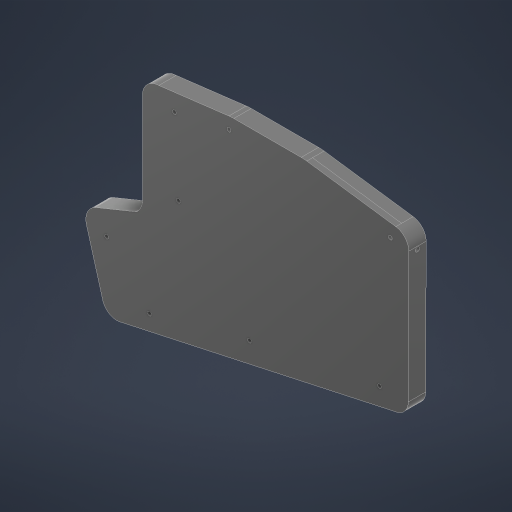
# Autodesk Inventor part: Case Bottom
Saved by Autodesk Inventor 2024.3 (Build 283343000, 343)
## iProperties
Created: 2024-12-13
Part Number: Case Bottom
Material: Generic
Document SubType Name: Modeling
Designer: micha
Density: 1 g/cm^3
Appearance: Smooth - Black
Author: micha
Autodesk Inventor part; units mm, degrees
ref_plane "YZ Plane" through (0, 0, 0) normal (1, 0, 0) x (0, 1, 0)
ref_plane "XZ Plane" through (0, 0, 0) normal (0, 1, 0) x (-1, 0, 0)
ref_plane "XY Plane" through (0, 0, 0) normal (0, 0, 1) x (1, 0, 0)
sketch "Sketch1" plane through (0, 0, 0) normal (0, 0, 1) x (1, 0, 0)
  arc A0 (-212.539, -59.4694) -> (-218.5045, -64.8588) centre (-212.5401, -65.4644) ccw projected
  line L0 (-174.0364, -54.7609) -> (-212.539, -59.4694) projected
  arc A1 (-171.7239, -54.62) -> (-174.0364, -54.7609) centre (-171.7239, -73.6702) ccw projected
  line L1 (-134.8832, -54.62) -> (-171.7239, -54.62) projected
  arc A2 (-132.2802, -54.7987) -> (-134.8832, -54.62) centre (-134.8832, -73.6711) ccw projected
  line L2 (-83.5422, -61.5211) -> (-132.2802, -54.7987) projected
  arc A3 (-79.23, -66.4736) -> (-83.5422, -61.5211) centre (-84.23, -66.4736) ccw projected
  line L3 (-79.4773, -138.0224) -> (-79.23, -66.4736) projected
  arc A4 (-82.9877, -142.7953) -> (-79.4773, -138.0224) centre (-84.4773, -138.0223) ccw projected
  line L4 (-234.3607, -175.7237) -> (-82.9877, -142.7953) projected
  arc A5 (-240.2338, -172.8773) -> (-234.3607, -175.7237) centre (-235.7454, -171.0986) ccw projected
  line L5 (-249.3284, -140.9769) -> (-240.2338, -172.8773) projected
  arc A6 (-246.2558, -134.3964) -> (-249.3284, -140.9769) centre (-243.557, -139.6641) ccw projected
  line L6 (-224.2532, -125.4096) -> (-246.2558, -134.3964) projected
  arc A7 (-224.2532, -125.4096) -> (-221.4228, -123.1302) centre (-226.6543, -119.531) ccw projected
  line L7 (-220.6818, -122.0531) -> (-221.4228, -123.1302) projected
  arc A8 (-220.6818, -122.0531) -> (-218.4447, -114.8395) centre (-231.1445, -114.8548) ccw projected
  line L8 (-218.5045, -64.8588) -> (-218.4447, -114.8395) projected
  circle A9 centre (-163.195, -152.4) radius 1.05 projected
  circle A10 centre (-92.075, -138.43) radius 1.05 projected
  circle A11 centre (-86.11, -127.04) radius 0.8509 projected
  circle A12 centre (-91.61, -127.04) radius 1.7145 projected
  circle A13 centre (-97.11, -127.04) radius 0.8509 projected
  circle A14 centre (-104.11, -127.04) radius 0.8509 projected
  circle A15 centre (-122.11, -139.04) radius 0.8509 projected
  circle A16 centre (-122.61, -135.29) radius 1.5 projected
  circle A17 centre (-109.61, -127.04) radius 1.7145 projected
  circle A18 centre (-115.11, -127.04) radius 0.8509 projected
  circle A19 centre (-86.61, -123.29) radius 1.5 projected
  circle A20 centre (-91.61, -121.09) radius 1.5 projected
  circle A21 centre (-96.61, -123.29) radius 1.5 projected
  circle A22 centre (-104.61, -123.29) radius 1.5 projected
  circle A23 centre (-109.61, -121.09) radius 1.5 projected
  circle A24 centre (-114.61, -123.29) radius 1.5 projected
  circle A25 centre (-122.11, -122.04) radius 0.8509 projected
  circle A26 centre (-122.61, -118.29) radius 1.5 projected
  circle A27 centre (-127.61, -139.04) radius 1.7145 projected
  circle A28 centre (-133.11, -139.04) radius 0.8509 projected
  circle A29 centre (-132.61, -135.29) radius 1.5 projected
  circle A30 centre (-140.11, -136.54) radius 0.8509 projected
  circle A31 centre (-127.61, -133.09) radius 1.5 projected
  circle A32 centre (-140.61, -132.79) radius 1.5 projected
  circle A33 centre (-145.61, -136.54) radius 1.7145 projected
  circle A34 centre (-151.11, -136.54) radius 0.8509 projected
  circle A35 centre (-158.11, -139.04) radius 0.8509 projected
  circle A36 centre (-163.61, -139.04) radius 1.7145 projected
  circle A37 centre (-158.61, -135.29) radius 1.5 projected
  circle A38 centre (-145.61, -130.59) radius 1.5 projected
  circle A39 centre (-150.61, -132.79) radius 1.5 projected
  circle A40 centre (-163.61, -133.09) radius 1.5 projected
  circle A41 centre (-127.61, -122.04) radius 1.7145 projected
  circle A42 centre (-133.11, -122.04) radius 0.8509 projected
  circle A43 centre (-140.11, -119.54) radius 0.8509 projected
  circle A44 centre (-127.61, -116.09) radius 1.5 projected
  circle A45 centre (-132.61, -118.29) radius 1.5 projected
  circle A46 centre (-140.61, -115.79) radius 1.5 projected
  circle A47 centre (-145.61, -119.54) radius 1.7145 projected
  circle A48 centre (-151.11, -119.54) radius 0.8509 projected
  circle A49 centre (-158.11, -122.04) radius 0.8509 projected
  circle A50 centre (-163.61, -122.04) radius 1.7145 projected
  circle A51 centre (-145.61, -113.59) radius 1.5 projected
  circle A52 centre (-150.61, -115.79) radius 1.5 projected
  circle A53 centre (-158.61, -118.29) radius 1.5 projected
  circle A54 centre (-163.61, -116.09) radius 1.5 projected
  circle A55 centre (-198.2508, -148.0493) radius 0.8509 projected
  circle A56 centre (-187.9141, -144.2871) radius 0.8509 projected
  circle A57 centre (-193.0824, -146.1682) radius 1.7145 projected
  circle A58 centre (-189.6666, -140.9342) radius 1.5 projected
  circle A59 centre (-199.0635, -144.3544) radius 1.5 projected
  circle A60 centre (-195.1175, -140.577) radius 1.5 projected
  circle A61 centre (-217.8966, -166.9609) radius 1.05 projected
  circle A62 centre (-217.2795, -154.9752) radius 0.8509 projected
  circle A63 centre (-236.3083, -161.9011) radius 0.8509 projected
  circle A64 centre (-225.9717, -158.1389) radius 0.8509 projected
  circle A65 centre (-231.14, -160.02) radius 1.7145 projected
  circle A66 centre (-227.7241, -154.7861) radius 1.5 projected
  circle A67 centre (-237.121, -158.2063) radius 1.5 projected
  circle A68 centre (-233.175, -154.4288) radius 1.5 projected
  circle A69 centre (-206.9429, -151.213) radius 0.8509 projected
  circle A70 centre (-212.1112, -153.0941) radius 1.7145 projected
  circle A71 centre (-208.6953, -147.8601) radius 1.5 projected
  circle A72 centre (-218.0923, -151.2803) radius 1.5 projected
  circle A73 centre (-214.1462, -147.5029) radius 1.5 projected
  circle A74 centre (-241.3, -142.24) radius 1.05 projected
  circle A75 centre (-169.11, -139.04) radius 0.8509 projected
  circle A76 centre (-168.61, -135.29) radius 1.5 projected
  circle A77 centre (-201.8629, -128.353) radius 0.8509 projected
  circle A78 centre (-169.11, -122.04) radius 0.8509 projected
  circle A79 centre (-176.11, -124.54) radius 0.8509 projected
  circle A80 centre (-181.61, -124.54) radius 1.7145 projected
  circle A81 centre (-176.61, -120.79) radius 1.5 projected
  circle A82 centre (-168.61, -118.29) radius 1.5 projected
  circle A83 centre (-181.61, -118.59) radius 1.5 projected
  circle A84 centre (-187.11, -124.54) radius 0.8509 projected
  circle A85 centre (-186.61, -120.79) radius 1.5 projected
  circle A86 centre (-194.5006, -125.0592) radius 0.4 projected
  circle A87 centre (-194.5006, -123.0592) radius 0.381 projected
  circle A88 centre (-194.5006, -121.0592) radius 0.381 projected
  circle A89 centre (-201.3506, -114.2092) radius 0.4 projected
  circle A90 centre (-220.8917, -135.2789) radius 0.8509 projected
  circle A91 centre (-207.0312, -130.2341) radius 1.7145 projected
  circle A92 centre (-212.1995, -132.1152) radius 0.8509 projected
  circle A93 centre (-222.6441, -131.9261) radius 1.5 projected
  circle A94 centre (-213.0123, -128.4203) radius 1.5 projected
  circle A95 centre (-226.06, -137.16) radius 1.7145 projected
  circle A96 centre (-231.2283, -139.0411) radius 0.8509 projected
  circle A97 centre (-232.041, -135.3463) radius 1.5 projected
  circle A98 centre (-228.095, -131.5688) radius 1.5 projected
  circle A99 centre (-203.6153, -125.0001) radius 1.5 projected
  circle A100 centre (-209.0662, -124.6429) radius 1.5 projected
  circle A101 centre (-203.3506, -114.2092) radius 0.4 projected
  circle A102 centre (-205.3506, -114.2092) radius 0.4 projected
  circle A103 centre (-86.11, -110.04) radius 0.8509 projected
  circle A104 centre (-91.61, -110.04) radius 1.7145 projected
  circle A105 centre (-86.61, -106.29) radius 1.5 projected
  circle A106 centre (-97.11, -110.04) radius 0.8509 projected
  circle A107 centre (-104.11, -110.04) radius 0.8509 projected
  circle A108 centre (-96.61, -106.29) radius 1.5 projected
  circle A109 centre (-104.61, -106.29) radius 1.5 projected
  circle A110 centre (-91.61, -104.09) radius 1.5 projected
  circle A111 centre (-109.61, -110.04) radius 1.7145 projected
  circle A112 centre (-115.11, -110.04) radius 0.8509 projected
  circle A113 centre (-114.61, -106.29) radius 1.5 projected
  circle A114 centre (-109.61, -104.09) radius 1.5 projected
  circle A115 centre (-122.11, -105.04) radius 0.8509 projected
  circle A116 centre (-122.61, -101.29) radius 1.5 projected
  circle A117 centre (-86.11, -93.04) radius 0.8509 projected
  circle A118 centre (-91.61, -93.04) radius 1.7145 projected
  circle A119 centre (-97.11, -93.04) radius 0.8509 projected
  circle A120 centre (-104.11, -93.04) radius 0.8509 projected
  circle A121 centre (-86.61, -89.29) radius 1.5 projected
  circle A122 centre (-91.61, -87.09) radius 1.5 projected
  circle A123 centre (-96.61, -89.29) radius 1.5 projected
  circle A124 centre (-104.61, -89.29) radius 1.5 projected
  circle A125 centre (-109.61, -93.04) radius 1.7145 projected
  circle A126 centre (-115.11, -93.04) radius 0.8509 projected
  circle A127 centre (-109.61, -87.09) radius 1.5 projected
  circle A128 centre (-114.61, -89.29) radius 1.5 projected
  circle A129 centre (-122.11, -88.04) radius 0.8509 projected
  circle A130 centre (-127.61, -105.04) radius 1.7145 projected
  circle A131 centre (-133.11, -105.04) radius 0.8509 projected
  circle A132 centre (-127.61, -99.09) radius 1.5 projected
  circle A133 centre (-132.61, -101.29) radius 1.5 projected
  circle A134 centre (-140.11, -102.54) radius 0.8509 projected
  circle A135 centre (-140.61, -98.79) radius 1.5 projected
  circle A136 centre (-145.61, -102.54) radius 1.7145 projected
  circle A137 centre (-151.11, -102.54) radius 0.8509 projected
  circle A138 centre (-150.61, -98.79) radius 1.5 projected
  circle A139 centre (-158.11, -105.04) radius 0.8509 projected
  circle A140 centre (-163.61, -105.04) radius 1.7145 projected
  circle A141 centre (-158.61, -101.29) radius 1.5 projected
  circle A142 centre (-163.61, -99.09) radius 1.5 projected
  circle A143 centre (-127.61, -88.04) radius 1.7145 projected
  circle A144 centre (-133.11, -88.04) radius 0.8509 projected
  circle A145 centre (-140.11, -85.54) radius 0.8509 projected
  circle A146 centre (-145.61, -96.59) radius 1.5 projected
  circle A147 centre (-145.61, -85.54) radius 1.7145 projected
  circle A148 centre (-151.11, -85.54) radius 0.8509 projected
  circle A149 centre (-158.11, -88.04) radius 0.8509 projected
  circle A150 centre (-163.61, -88.04) radius 1.7145 projected
  circle A151 centre (-86.11, -76.04) radius 0.8509 projected
  circle A152 centre (-91.61, -76.04) radius 1.7145 projected
  circle A153 centre (-86.61, -72.29) radius 1.5 projected
  circle A154 centre (-97.11, -76.04) radius 0.8509 projected
  circle A155 centre (-104.11, -76.04) radius 0.8509 projected
  circle A156 centre (-96.61, -72.29) radius 1.5 projected
  circle A157 centre (-104.61, -72.29) radius 1.5 projected
  circle A158 centre (-122.61, -84.29) radius 1.5 projected
  circle A159 centre (-109.61, -76.04) radius 1.7145 projected
  circle A160 centre (-115.11, -76.04) radius 0.8509 projected
  circle A161 centre (-114.61, -72.29) radius 1.5 projected
  circle A162 centre (-122.11, -71.04) radius 0.8509 projected
  circle A163 centre (-91.61, -70.09) radius 1.5 projected
  circle A164 centre (-86.1194, -65.1034) radius 1.05 projected
  circle A165 centre (-109.61, -70.09) radius 1.5 projected
  circle A166 centre (-122.61, -67.29) radius 1.5 projected
  circle A167 centre (-127.61, -82.09) radius 1.5 projected
  circle A168 centre (-132.61, -84.29) radius 1.5 projected
  circle A169 centre (-140.61, -81.79) radius 1.5 projected
  circle A170 centre (-127.61, -71.04) radius 1.7145 projected
  circle A171 centre (-133.11, -71.04) radius 0.8509 projected
  circle A172 centre (-150.61, -81.79) radius 1.5 projected
  circle A173 centre (-145.61, -79.59) radius 1.5 projected
  circle A174 centre (-158.61, -84.29) radius 1.5 projected
  circle A175 centre (-163.61, -82.09) radius 1.5 projected
  circle A176 centre (-158.11, -71.04) radius 0.8509 projected
  circle A177 centre (-163.61, -71.04) radius 1.7145 projected
  circle A178 centre (-127.61, -65.09) radius 1.5 projected
  circle A179 centre (-132.61, -67.29) radius 1.5 projected
  circle A180 centre (-140.11, -68.54) radius 0.8509 projected
  circle A181 centre (-140.61, -64.79) radius 1.5 projected
  circle A182 centre (-145.61, -68.54) radius 1.7145 projected
  circle A183 centre (-151.11, -68.54) radius 0.8509 projected
  circle A184 centre (-150.61, -64.79) radius 1.5 projected
  circle A185 centre (-158.61, -67.29) radius 1.5 projected
  circle A186 centre (-163.61, -65.09) radius 1.5 projected
  circle A187 centre (-145.61, -62.59) radius 1.5 projected
  circle A188 centre (-176.11, -107.54) radius 0.8509 projected
  circle A189 centre (-181.61, -107.54) radius 1.7145 projected
  circle A190 centre (-169.11, -105.04) radius 0.8509 projected
  circle A191 centre (-168.61, -101.29) radius 1.5 projected
  circle A192 centre (-176.61, -103.79) radius 1.5 projected
  circle A193 centre (-181.61, -101.59) radius 1.5 projected
  circle A194 centre (-187.11, -107.54) radius 0.8509 projected
  circle A195 centre (-202.0465, -105.6044) radius 1.05 projected
  circle A196 centre (-186.61, -103.79) radius 1.5 projected
  circle A197 centre (-169.11, -88.04) radius 0.8509 projected
  circle A198 centre (-176.11, -90.54) radius 0.8509 projected
  circle A199 centre (-181.61, -90.54) radius 1.7145 projected
  circle A200 centre (-176.61, -86.79) radius 1.5 projected
  circle A201 centre (-195.58, -92.9563) radius 0.5461 projected
  circle A202 centre (-187.11, -90.54) radius 0.8509 projected
  circle A203 centre (-186.61, -86.79) radius 1.5 projected
  circle A204 centre (-195.58, -90.4163) radius 0.5461 projected
  circle A205 centre (-195.58, -87.8763) radius 0.5461 projected
  circle A206 centre (-195.58, -85.3363) radius 0.5461 projected
  arc A207 (-207.5558, -104.4294) -> (-207.5558, -103.5294) centre (-207.5558, -103.9794) ccw projected
  line L9 (-207.5558, -103.5294) -> (-208.1558, -103.5294) projected
  arc A208 (-208.1558, -103.5294) -> (-208.1558, -104.4294) centre (-208.1558, -103.9794) ccw projected
  line L10 (-208.1558, -104.4294) -> (-207.5558, -104.4294) projected
  arc A209 (-211.5558, -104.4294) -> (-211.5558, -103.5294) centre (-211.5558, -103.9794) ccw projected
  line L11 (-211.5558, -103.5294) -> (-212.1558, -103.5294) projected
  arc A210 (-212.1558, -103.5294) -> (-212.1558, -104.4294) centre (-212.1558, -103.9794) ccw projected
  line L12 (-212.1558, -104.4294) -> (-211.5558, -104.4294) projected
  arc A211 (-206.4558, -102.1294) -> (-206.4558, -101.2294) centre (-206.4558, -101.6794) ccw projected
  line L13 (-206.4558, -101.2294) -> (-207.0558, -101.2294) projected
  arc A212 (-207.0558, -101.2294) -> (-207.0558, -102.1294) centre (-207.0558, -101.6794) ccw projected
  line L14 (-207.0558, -102.1294) -> (-206.4558, -102.1294) projected
  arc A213 (-206.4558, -99.8294) -> (-206.4558, -98.9294) centre (-206.4558, -99.3794) ccw projected
  line L15 (-206.4558, -98.9294) -> (-207.0558, -98.9294) projected
  arc A214 (-207.0558, -98.9294) -> (-207.0558, -99.8294) centre (-207.0558, -99.3794) ccw projected
  line L16 (-207.0558, -99.8294) -> (-206.4558, -99.8294) projected
  circle A215 centre (-209.4558, -101.6794) radius 0.75 projected
  circle A216 centre (-209.4558, -99.3794) radius 0.75 projected
  arc A217 (-214.5558, -104.4294) -> (-214.5558, -103.5294) centre (-214.5558, -103.9794) ccw projected
  line L17 (-214.5558, -103.5294) -> (-215.1558, -103.5294) projected
  arc A218 (-215.1558, -103.5294) -> (-215.1558, -104.4294) centre (-215.1558, -103.9794) ccw projected
  line L18 (-215.1558, -104.4294) -> (-214.5558, -104.4294) projected
  circle A219 centre (-216.4558, -101.6794) radius 0.75 projected
  circle A220 centre (-216.4558, -99.3794) radius 0.75 projected
  arc A221 (-207.5558, -97.5294) -> (-207.5558, -96.6294) centre (-207.5558, -97.0794) ccw projected
  line L19 (-207.5558, -96.6294) -> (-208.1558, -96.6294) projected
  arc A222 (-208.1558, -96.6294) -> (-208.1558, -97.5294) centre (-208.1558, -97.0794) ccw projected
  line L20 (-208.1558, -97.5294) -> (-207.5558, -97.5294) projected
  arc A223 (-211.5558, -97.5294) -> (-211.5558, -96.6294) centre (-211.5558, -97.0794) ccw projected
  line L21 (-211.5558, -96.6294) -> (-212.1558, -96.6294) projected
  arc A224 (-212.1558, -96.6294) -> (-212.1558, -97.5294) centre (-212.1558, -97.0794) ccw projected
  line L22 (-212.1558, -97.5294) -> (-211.5558, -97.5294) projected
  circle A225 centre (-210.82, -92.9563) radius 0.5461 projected
  arc A226 (-214.5558, -97.5294) -> (-214.5558, -96.6294) centre (-214.5558, -97.0794) ccw projected
  line L23 (-214.5558, -96.6294) -> (-215.1558, -96.6294) projected
  arc A227 (-215.1558, -96.6294) -> (-215.1558, -97.5294) centre (-215.1558, -97.0794) ccw projected
  line L24 (-215.1558, -97.5294) -> (-214.5558, -97.5294) projected
  circle A228 centre (-210.82, -90.4163) radius 0.5461 projected
  circle A229 centre (-210.82, -87.8763) radius 0.5461 projected
  circle A230 centre (-210.82, -85.3363) radius 0.5461 projected
  circle A231 centre (-168.61, -84.29) radius 1.5 projected
  circle A232 centre (-181.61, -84.59) radius 1.5 projected
  circle A233 centre (-169.11, -71.04) radius 0.8509 projected
  circle A234 centre (-176.11, -73.54) radius 0.8509 projected
  circle A235 centre (-181.61, -73.54) radius 1.7145 projected
  circle A236 centre (-195.58, -82.7963) radius 0.5461 projected
  circle A237 centre (-195.58, -80.2563) radius 0.5461 projected
  circle A238 centre (-187.11, -73.54) radius 0.8509 projected
  circle A239 centre (-195.58, -77.7163) radius 0.5461 projected
  circle A240 centre (-195.58, -75.1763) radius 0.5461 projected
  circle A241 centre (-199.5, -77.7363) radius 0.2 projected
  circle A242 centre (-199.45, -75.2863) radius 0.2 projected
  circle A243 centre (-195.58, -72.6363) radius 0.5461 projected
  circle A244 centre (-199.45, -72.6363) radius 0.2 projected
  circle A245 centre (-168.61, -67.29) radius 1.5 projected
  circle A246 centre (-176.61, -69.79) radius 1.5 projected
  circle A247 centre (-181.61, -67.59) radius 1.5 projected
  circle A248 centre (-174.3426, -58.0743) radius 1.05 projected
  circle A249 centre (-186.61, -69.79) radius 1.5 projected
  circle A250 centre (-195.58, -70.0963) radius 0.5461 projected
  circle A251 centre (-195.58, -67.5563) radius 0.5461 projected
  circle A252 centre (-199.4864, -69.9863) radius 0.2 projected
  circle A253 centre (-195.58, -65.0163) radius 0.5461 projected
  circle A254 centre (-210.82, -82.7963) radius 0.5461 projected
  circle A255 centre (-210.82, -80.2563) radius 0.5461 projected
  circle A256 centre (-206.55, -77.7863) radius 0.2 projected
  circle A257 centre (-206.55, -75.2363) radius 0.2 projected
  circle A258 centre (-210.82, -77.7163) radius 0.5461 projected
  circle A259 centre (-210.82, -75.1763) radius 0.5461 projected
  circle A260 centre (-206.55, -72.6363) radius 0.2 projected
  circle A261 centre (-210.82, -72.6363) radius 0.5461 projected
  circle A262 centre (-206.55, -70.1863) radius 0.2 projected
  circle A263 centre (-210.82, -70.0963) radius 0.5461 projected
  circle A264 centre (-210.82, -67.5563) radius 0.5461 projected
  circle A265 centre (-204.2038, -64.7368) radius 1.05 projected
  circle A266 centre (-210.82, -65.0163) radius 0.5461 projected
  arc A267 (-212.7525, -56.2968) -> (-221.6632, -64.5381) centre (-212.5401, -65.4644) ccw
  line L25 (-212.7525, -56.2968) -> (-174.4218, -51.6093)
  arc A268 (-171.7239, -51.445) -> (-174.4218, -51.6093) centre (-171.7239, -73.6702) ccw
  line L26 (-171.7239, -51.445) -> (-134.8832, -51.445)
  arc A269 (-131.8463, -51.6535) -> (-134.8832, -51.445) centre (-134.8832, -73.6711) ccw
  line L27 (-131.8463, -51.6535) -> (-83.113, -58.3752)
  arc A270 (-76.055, -66.4797) -> (-83.113, -58.3752) centre (-84.23, -66.4736) ccw
  line L28 (-76.055, -66.4797) -> (-76.3023, -138.0285)
  arc A271 (-82.1926, -145.8716) -> (-76.3023, -138.0285) centre (-84.4773, -138.0223) ccw
  line L29 (-82.1926, -145.8716) -> (-233.5818, -178.8035)
  arc A272 (-243.2492, -173.8808) -> (-233.5818, -178.8035) centre (-235.7454, -171.0986) ccw
  line L30 (-243.2492, -173.8808) -> (-252.4027, -141.7737)
  arc A273 (-247.5689, -131.5031) -> (-252.4027, -141.7737) centre (-243.557, -139.6641) ccw
  line L31 (-247.5689, -131.5031) -> (-225.4538, -122.4703)
  arc A274 (-225.4538, -122.4703) -> (-224.0386, -121.3306) centre (-226.6543, -119.531) ccw
  line L32 (-224.0386, -121.3306) -> (-223.2975, -120.2534)
  arc A275 (-223.2975, -120.2534) -> (-221.6197, -114.8434) centre (-231.1445, -114.8548) ccw
  line L33 (-221.6197, -114.8434) -> (-221.6632, -78.4471)
  line L34 (-221.6632, -78.4471) -> (-221.6632, -64.5381)
  point P0 (0, 0)
  point P1 (-218.5045, -64.8588)
  dimension "d0" = 3.175
  constraints: 20 end point, 18 point on circle, 9 centre point, 1 vertical, 17 other
  measures "d0" distance between parallel lines of L3 L28
extrude "Extrusion1" add sketch "Sketch1" along normal blind 3.175 contours L0 A1 L1 A2 L2 A3 L3 A4 L4 A5 L5 A6 L6 A7 L7 A8 L8 A0 | A11 | A12 | A13 | A14 | A15 | A16 | A17 | A18 | A19 | A20 | A21 | A22 | A23 | A24 | A25 | A26 | A27 | A28 | A29 | A30 | A31 | A32 | A33 | A34 | A35 | A36 | A37 | A38 | A39 | A40 | A41 | A42 | A43 | A44 | A45 | A46 | A47 | A48 | A49 | A50 | A51 | A52 | A53 | A54 | A55 | A56 | A57 | A58 | A59 | A60 | A62 | A63 | A64 | A65 | A66 | A67 | A68 | A69 | A70 | A71 | A72 | A73 | A75 | A76 | A77 | A78 | A79 | A80 | A81 | A82 | A83 | A84 | A85 | A86 | A87 | A88 | A89 | A90 | A91 | A92 | A93 | A94 | A95 | A96 | A97 | A98 | A99 | A100 | A101 | A102 | A103 | A104 | A105 | A106 | A107 | A108 | A109 | A110 | A111 | A112 | A113 | A114 | A115 | A116 | A117 | A118 | A119 | A120 | A121 | A122 | A123 | A124 | A125 | A126 | A127 | A128 | A129 | A130 | A131 | A132 | A133 | A134 | A135 | A136 | A137 | A138 | A139 | A140 | A141 | A142 | A143 | A144 | A145 | A146 | A147 | A148 | A149 | A150 | A151 | A152 | A153 | A154 | A155 | A156 | A157 | A158 | A159 | A160 | A161 | A162 | A163 | A165 | A166 | A167 | A168 | A169 | A170 | A171 | A172 | A173 | A174 | A175 | A176 | A177 | A178 | A179 | A180 | A181 | A182 | A183 | A184 | A185 | A186 | A187 | A188 | A189 | A190 | A191 | A192 | A193 | A194 | A196 | A197 | A198 | A199 | A200 | A201 | A202 | A203 | A204 | A205 | A206 | L10 A208 L9 A207 | L12 A210 L11 A209 | L14 A212 L13 A211 | L16 A214 L15 A213 | A215 | A216 | L18 A218 L17 A217 | A219 | A220 | L20 A222 L19 A221 | L22 A224 L21 A223 | A225 | L24 A227 L23 A226 | A228 | A229 | A230 | A231 | A232 | A233 | A234 | A235 | A236 | A237 | A238 | A239 | A240 | A241 | A242 | A243 | A244 | A245 | A246 | A247 | A249 | A250 | A251 | A252 | A253 | A254 | A255 | A256 | A257 | A258 | A259 | A260 | A261 | A262 | A263 | A264 | A266 | L25 A268 L26 A269 L27 A270 L28 A271 L29 A272 L30 A273 L31 A274 L32 A275 L33 L34 A267
sketch "Sketch2" plane through (0, 0, 0) normal (0, 0, -1) x (-1, 0, 0)
  line L0 (174.4218, -51.6093) -> (212.7525, -56.2968) projected
  arc A0 (174.4218, -51.6093) -> (171.7239, -51.445) centre (171.7239, -73.6702) ccw projected
  line L1 (134.8832, -51.445) -> (171.7239, -51.445) projected
  arc A1 (134.8832, -51.445) -> (131.8463, -51.6535) centre (134.8832, -73.6711) ccw projected
  line L2 (83.113, -58.3752) -> (131.8463, -51.6535) projected
  arc A2 (83.113, -58.3752) -> (76.055, -66.4797) centre (84.23, -66.4736) ccw projected
  line L3 (76.3023, -138.0285) -> (76.055, -66.4797) projected
  arc A3 (76.3023, -138.0285) -> (82.1926, -145.8716) centre (84.4773, -138.0223) ccw projected
  line L4 (233.5818, -178.8035) -> (82.1926, -145.8716) projected
  arc A4 (233.5818, -178.8035) -> (243.2492, -173.8808) centre (235.7454, -171.0986) ccw projected
  line L5 (252.4027, -141.7737) -> (243.2492, -173.8808) projected
  arc A5 (252.4027, -141.7737) -> (247.5689, -131.5031) centre (243.557, -139.6641) ccw projected
  line L6 (225.4538, -122.4703) -> (247.5689, -131.5031) projected
  arc A6 (224.0386, -121.3306) -> (225.4538, -122.4703) centre (226.6543, -119.531) ccw projected
  line L7 (223.2975, -120.2534) -> (224.0386, -121.3306) projected
  arc A7 (221.6197, -114.8434) -> (223.2975, -120.2534) centre (231.1445, -114.8548) ccw projected
  line L8 (221.6632, -78.4471) -> (221.6197, -114.8434) projected
  line L9 (221.6632, -64.5381) -> (221.6632, -78.4471) projected
  arc A8 (221.6632, -64.5381) -> (212.7525, -56.2968) centre (212.5401, -65.4644) ccw projected
  line L10 (212.5468, -59.3424) -> (174.0518, -54.6348)
  arc A9 (174.0518, -54.6348) -> (171.7239, -54.493) centre (171.7239, -73.6702) ccw
  line L11 (171.7239, -54.493) -> (134.8832, -54.493)
  arc A10 (134.8832, -54.493) -> (132.2628, -54.6729) centre (134.8832, -73.6711) ccw
  line L12 (132.2628, -54.6729) -> (83.5295, -61.3946)
  arc A11 (83.5295, -61.3946) -> (79.103, -66.4738) centre (84.23, -66.4736) ccw
  line L13 (79.103, -66.4738) -> (79.3503, -138.0226)
  arc A12 (79.3503, -138.0226) -> (82.9553, -142.9182) centre (84.4773, -138.0223) ccw
  line L14 (82.9553, -142.9182) -> (234.329, -175.8468)
  arc A13 (234.329, -175.8468) -> (240.3542, -172.9182) centre (235.7454, -171.0986) ccw
  line L15 (240.3542, -172.9182) -> (249.4514, -141.0084)
  arc A14 (249.4514, -141.0084) -> (246.3088, -134.2809) centre (243.557, -139.6641) ccw
  line L16 (246.3088, -134.2809) -> (224.3013, -125.292)
  arc A15 (221.5274, -123.0582) -> (224.3013, -125.292) centre (226.6543, -119.531) ccw
  line L17 (221.5274, -123.0582) -> (220.7864, -121.9811)
  arc A16 (218.5717, -114.8398) -> (220.7864, -121.9811) centre (231.1445, -114.8548) ccw
  line L18 (218.5717, -114.8398) -> (218.6152, -78.4453)
  line L19 (218.6152, -78.4453) -> (218.6152, -64.708)
  arc A17 (218.6152, -64.708) -> (212.5468, -59.3424) centre (212.5401, -65.4644) ccw
  point P0 (0, 0)
  dimension "d3" = 3.048
  constraints: 20 end point, 18 point on circle, 9 centre point, 18 other
  measures "d3" distance between parallel lines of L0 L10
extrude "Extrusion2" add sketch "Sketch2" along normal blind 6.35
sketch "Sketch3" plane through (0, 0, 0) normal (0, 0, -1) x (-1, 0, 0)
  circle A0 centre (131.8463, -59.1243) radius 1.5875
  circle A1 centre (86.1194, -65.1034) radius 1.05 projected
  line L0 (174.4218, -51.6093) -> (212.7525, -56.2968) projected
  arc A2 (221.6632, -64.5381) -> (212.7525, -56.2968) centre (212.5401, -65.4644) ccw projected
  line L1 (221.6632, -64.5381) -> (221.6632, -78.4471) projected
  line L2 (221.6632, -78.4471) -> (221.6197, -114.8434) projected
  arc A3 (221.6197, -114.8434) -> (223.2975, -120.2534) centre (231.1445, -114.8548) ccw projected
  line L3 (223.2975, -120.2534) -> (224.0386, -121.3306) projected
  arc A4 (224.0386, -121.3306) -> (225.4538, -122.4703) centre (226.6543, -119.531) ccw projected
  line L4 (225.4538, -122.4703) -> (247.5689, -131.5031) projected
  arc A5 (252.4027, -141.7737) -> (247.5689, -131.5031) centre (243.557, -139.6641) ccw projected
  line L5 (252.4027, -141.7737) -> (243.2492, -173.8808) projected
  arc A6 (233.5818, -178.8035) -> (243.2492, -173.8808) centre (235.7454, -171.0986) ccw projected
  line L6 (233.5818, -178.8035) -> (82.1926, -145.8716) projected
  arc A7 (76.3023, -138.0285) -> (82.1926, -145.8716) centre (84.4773, -138.0223) ccw projected
  line L7 (76.3023, -138.0285) -> (76.055, -66.4797) projected
  arc A8 (83.113, -58.3752) -> (76.055, -66.4797) centre (84.23, -66.4736) ccw projected
  line L8 (83.113, -58.3752) -> (131.8463, -51.6535) projected
  arc A9 (134.8832, -51.445) -> (131.8463, -51.6535) centre (134.8832, -73.6711) ccw projected
  line L9 (134.8832, -51.445) -> (171.7239, -51.445) projected
  arc A10 (174.4218, -51.6093) -> (171.7239, -51.445) centre (171.7239, -73.6702) ccw projected
  circle A11 centre (202.0465, -105.6044) radius 1.05 projected
  circle A12 centre (92.075, -138.43) radius 1.05 projected
  circle A13 centre (86.1194, -65.1034) radius 1.05 projected
  circle A14 centre (204.2038, -64.7368) radius 1.05 projected
  circle A15 centre (174.3426, -58.0743) radius 1.05 projected
  circle A16 centre (241.3, -142.24) radius 1.05 projected
  circle A17 centre (217.8966, -166.9609) radius 1.05 projected
  circle A18 centre (163.195, -152.4) radius 1.05 projected
  circle A19 centre (86.1194, -65.1034) radius 1.8438
  circle A20 centre (92.075, -138.43) radius 1.8438
  circle A21 centre (163.195, -152.4) radius 1.8438
  circle A22 centre (217.8966, -166.9609) radius 1.8438
  circle A23 centre (241.3, -142.24) radius 1.8438
  circle A24 centre (202.0465, -105.6044) radius 1.8438
  circle A25 centre (204.2038, -64.7368) radius 1.8438
  circle A26 centre (174.3426, -58.0743) radius 1.8438
  circle A27 centre (102.0786, -82.6755) radius 1.5875
  circle A28 centre (145.7141, -74.7536) radius 1.5875
  circle A29 centre (177.6615, -81.088) radius 1.5875
  circle A30 centre (203.1538, -86.052) radius 1.5875
  circle A31 centre (177.6615, -96.6453) radius 1.5875
  circle A32 centre (145.7141, -90.8571) radius 1.5875
  circle A33 centre (101.8189, -100.2076) radius 1.5875
  circle A34 centre (101.8189, -116.0514) radius 1.5875
  circle A35 centre (145.7141, -108.9087) radius 1.5875
  circle A36 centre (177.6615, -114.4639) radius 1.5875
  circle A37 centre (137.922, -126.9867) radius 1.5875
  circle A38 centre (171.7051, -130.3369) radius 1.5875
  circle A39 centre (205.2538, -139.6025) radius 1.5875
  circle A40 centre (187.921, -151.35) radius 1.5875
  circle A41 centre (86.1194, -65.1034) radius 0.9738
  circle A42 centre (174.3426, -58.0743) radius 0.9738
  circle A43 centre (204.2038, -64.7368) radius 0.9738
  circle A44 centre (202.0465, -105.6044) radius 0.9738
  circle A45 centre (241.3, -142.24) radius 0.9738
  circle A46 centre (217.8966, -166.9609) radius 0.9738
  circle A47 centre (163.195, -152.4) radius 0.9738
  circle A48 centre (92.075, -138.43) radius 0.9738
  point P0 (0, 0)
  dimension "d6" = 3.175
  dimension "d7" = 0.7937
  dimension "d8" = 0.7937
  dimension "d9" = 0.7937
  dimension "d10" = 0.7937
  dimension "d11" = 0.7937
  dimension "d12" = 0.7937
  dimension "d13" = 0.7937
  dimension "d14" = 0.7937
  dimension "d15" = 3.175
  dimension "d16" = 3.175
  dimension "d17" = 3.175
  dimension "d18" = 3.175
  dimension "d19" = 3.175
  dimension "d20" = 3.175
  dimension "d21" = 3.175
  dimension "d22" = 3.175
  dimension "d23" = 3.175
  dimension "d24" = 3.175
  dimension "d25" = 3.175
  dimension "d26" = 3.175
  dimension "d27" = 3.175
  dimension "d28" = 3.175
  dimension "d46" = 0.0762
  dimension "d47" = 0.0762
  dimension "d48" = 0.0762
  dimension "d49" = 0.0762
  dimension "d50" = 0.0762
  dimension "d51" = 0.0762
  dimension "d52" = 0.0762
  dimension "d53" = 0.0762
  constraints: 31 centre point
  measures "d6" diameter of A0
  measures "d7" radial gap between concentric circles of A1 A19
  measures "d8" radial gap between concentric circles of A12 A20
  measures "d9" radial gap between concentric circles of A18 A21
  measures "d10" radial gap between concentric circles of A17 A22
  measures "d11" radial gap between concentric circles of A16 A23
  measures "d12" radial gap between concentric circles of A11 A24
  measures "d13" radial gap between concentric circles of A14 A25
  measures "d14" radial gap between concentric circles of A15 A26
  measures "d15" diameter of A27
  measures "d16" diameter of A28
  measures "d17" diameter of A29
  measures "d18" diameter of A30
  measures "d19" diameter of A31
  measures "d20" diameter of A32
  measures "d21" diameter of A33
  measures "d22" diameter of A34
  measures "d23" diameter of A35
  measures "d24" diameter of A36
  measures "d25" diameter of A37
  measures "d26" diameter of A38
  measures "d27" diameter of A39
  measures "d28" diameter of A40
  measures "d46" radial gap between concentric circles of A1 A41
  measures "d47" radial gap between concentric circles of A15 A42
  measures "d48" radial gap between concentric circles of A14 A43
  measures "d49" radial gap between concentric circles of A11 A44
  measures "d50" radial gap between concentric circles of A16 A45
  measures "d51" radial gap between concentric circles of A17 A46
  measures "d52" radial gap between concentric circles of A18 A47
  measures "d53" radial gap between concentric circles of A12 A48
extrude "Extrusion3" add sketch "Sketch3" along normal blind 3.175 contours A1 | A11 | A12 | A14 | A15 | A16 | A17 | A18 | A19 | A20 | A21 | A22 | A23 | A24 | A25 | A26 | A27 | A28 | A29 | A30 | A31 | A32 | A33 | A34 | A35 | A36 | A37 | A38 | A39 | A40
sketch "Sketch4" plane through (-218.6152, -78.4453, 0) normal (1, 0, 0) x (0, 0, -1)
  line L0 (0, 0) -> (0, 13.7373) projected
  line L1 (0, 0) -> (6.35, 0) projected
  line L2 (6.35, 13.7373) -> (6.35, 0) projected
  line L3 (0, 13.7373) -> (6.35, 13.7373) projected
  circle A0 centre (1.5875, 12.1498) radius 1.1906
  point P0 (0, 78.4453)
  dimension "d31" = 2.3813
  dimension "d32" = 1.5875
  dimension "d33" = 4.7625
  constraints: 1 centre point
  measures "d31" diameter of A0
  measures "d32" distance from line of L3 A0.centre
  measures "d33" distance from line of L2 A0.centre
sketch "Sketch5" plane through (-79.103, -66.4738, -6.35) normal (-0.999994, 0.0034561, 0) x (0, 0, 1)
  line L0 (6.35, 0) -> (6.35, -71.5492) projected
  line L1 (6.35, 0) -> (0, 0) projected
  line L2 (0, -71.5492) -> (0, 0) projected
  line L3 (6.35, -71.5492) -> (0, -71.5492) projected
  circle A0 centre (4.7625, -1.5875) radius 1.1906
  point P0 (6.35, 66.7468)
  dimension "d34" = 2.3813
  dimension "d35" = 4.7625
  dimension "d36" = 1.5875
  constraints: 1 centre point
  measures "d34" diameter of A0
  measures "d35" distance from line of L2 A0.centre
  measures "d36" distance from line of L1 A0.centre
sketch "Sketch6" plane through (-240.3542, -172.9182, 0) normal (0.9616814, 0.2741696, 0) x (0, 0, -1)
  line L0 (0, 0) -> (0, 33.1812) projected
  line L1 (0, 0) -> (6.35, 0) projected
  line L2 (6.35, 33.1812) -> (6.35, 0) projected
  line L3 (0, 33.1812) -> (6.35, 33.1812) projected
  circle A0 centre (1.5875, 25.2437) radius 1.1906
  point P0 (0, 100.3944)
  dimension "d37" = 2.3813
  dimension "d38" = 4.7625
  dimension "d39" = 7.9375
  constraints: 1 centre point
  measures "d37" diameter of A0
  measures "d38" distance from line of L2 A0.centre
  measures "d39" distance from line of L3 A0.centre
extrude "Extrusion4" cut sketch "Sketch6" against normal blind 6.35 contours A0
extrude "Extrusion5" cut sketch "Sketch4" against normal blind 6.35 contours A0
extrude "Extrusion6" cut sketch "Sketch5" against normal blind 6.35 contours A0
equation "\"d8\" = d7"
equation "\"d9\" = d7"
equation "\"d10\" = d7"
equation "\"d11\" = d7"
equation "\"d12\" = d7"
equation "\"d13\" = d7"
equation "\"d14\" = d7"
equation "\"d34\" = d31"
equation "\"d37\" = d31"
body "Solid1"
